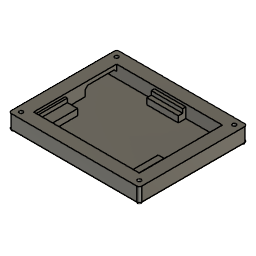
bottom (Autodesk Fusion 360 design; units mm, degrees)
part number: 2026-02-21-15-50-16-128
Autodesk Fusion 360 part; units mm, degrees
sketch "Schizzo1" plane through (0, 0, 0) normal (0, 0, 1) x (1, 0, 0)
  line L0 (0, 0) -> (84, 0)
  line L1 (84, 0) -> (84, 66)
  line L2 (84, 66) -> (0, 66)
  line L3 (0, 66) -> (0, 0)
  line L4 (-10, -10) -> (94, -10)
  line L5 (94, -10) -> (94, 76)
  line L6 (94, 76) -> (-10, 76)
  line L7 (-10, 76) -> (-10, -10)
  circle A0 centre (-5, 71) radius 1.45
  circle A1 centre (-5, -5) radius 1.45
  circle A2 centre (89, -5) radius 1.45
  circle A3 centre (88.5374, 71) radius 1.45
  line L8 (0, 66) -> (84, 66)
  line L9 (84, 66) -> (84, 0)
  line L10 (84, 0) -> (0, 0)
  line L11 (0, 0) -> (0, 66)
  dimension "d1" = 84
  dimension "d2" = 66
  dimension "d3" = 10
  dimension "d4" = 2.9
  dimension "d5" = 2.9
  dimension "d6" = 2.9
  dimension "d7" = 5
  dimension "d8" = 5
  dimension "d9" = 5
  dimension "d10" = 5
  dimension "d11" = 5
  dimension "d12" = 2.9
  dimension "d13" = 5
  dimension "d14" = 5.4626
  constraint horizontal L0
  constraint vertical L1
  constraint horizontal L2
  constraint vertical L3
  constraint coincident L0.start L3.end
  constraint horizontal L8
  constraint vertical L9
  constraint horizontal L10
  constraint vertical L11
  measures "d1" distance of L0.start L0.end
  measures "d2" distance of L0.start L2.end
  measures "d4" diameter of A0
  measures "d5" diameter of A1
  measures "d6" diameter of A2
  measures "d7" distance of L4 A2.centre
  measures "d8" distance of L5 A2.centre
  measures "d9" distance of L4 A1.centre
  measures "d10" distance of L6 A0.centre
  measures "d11" distance of L7 A0.centre
  measures "d12" diameter of A3
  measures "d13" distance of L6 A3.centre
  measures "d14" distance of L5 A3.centre
extrude "Estrusione1" add sketch "Schizzo1" along normal blind 13
sketch "Schizzo2" plane through (0, 0, 0) normal (0, 0, 1) x (1, 0, 0)
  line L0 (0, 0) -> (84, 0)
  line L1 (84, 0) -> (84, 66)
  line L2 (84, 66) -> (0, 66)
  line L3 (0, 66) -> (0, 0)
  constraint horizontal L0
  constraint vertical L1
  constraint horizontal L2
  constraint vertical L3
  constraint coincident L0.start L3.end
extrude "Estrusione2" add sketch "Schizzo2" along normal blind 3
sketch "Sketch3" plane through (-10, 0, 0) normal (-1, 0, 0) x (0, -1, 0)
  line L0 (-76, 0) -> (10, 0)
  line L1 (10, 0) -> (10, 13)
  line L2 (10, 13) -> (-76, 13)
  line L3 (-76, 13) -> (-76, 0)
  line L4 (-66, 3) -> (-41, 3)
  line L5 (-41, 3) -> (-41, 8)
  line L6 (-41, 8) -> (-43, 10)
  line L7 (-43, 10) -> (-64, 10)
  line L8 (-64, 10) -> (-66, 8)
  line L9 (-66, 8) -> (-66, 3)
  constraint horizontal L4
  constraint perpendicular L4 L5
  constraint perpendicular L5 L7
  constraint perpendicular L6 L8
  constraint perpendicular L4 L9
extrude "Extrude3" cut sketch "Sketch3" against normal blind 10 contours L4 L5 L6 L7 L8 L9
fillet "Fillet1" radius 2 4 edges at (94, 33, 0) (42, -10, 0) (-10, 33, 0) (42, 76, 0)
fillet "Fillet2" radius 2 8 edges at (-9.4142, -9.4142, 0.5858) (-10, -10, 7.5) (93.4142, -9.4142, 0.5858) (94, -10, 7.5) (93.4142, 75.4142, 0.5858) (94, 76, 7.5) (-9.4142, 75.4142, 0.5858) (-10, 76, 7.5)
sketch "Sketch4" plane through (0, 0, 3) normal (0, 0, 1) x (-1, 0, 0)
  line L0 (0, -41) -> (0, 0)
  line L1 (0, 0) -> (-84, 0)
  line L2 (-84, 0) -> (-84, -66)
  line L3 (-84, -66) -> (10, -66)
  line L4 (10, -66) -> (10, -41)
  line L5 (10, -41) -> (0, -41)
  line L6 (0, 0) -> (-10, 0)
  line L7 (-10, 0) -> (-10, -25)
  line L8 (-10, -25) -> (0, -25)
  line L9 (0, -25) -> (0, 0)
  constraint horizontal L6
  constraint vertical L7
  constraint horizontal L8
  constraint vertical L9
  constraint coincident L0.end L1.start
extrude "Extrude4" add sketch "Sketch4" along normal blind 5 contours L0 L1 L6 L7 L8 L9
sketch "Sketch5" plane through (0, 0, 3) normal (0, 0, 1) x (-1, 0, 0)
  line L0 (-10, -25) -> (-10, 0)
  line L1 (-10, 0) -> (-84, 0)
  line L2 (-84, 0) -> (-84, -66)
  line L3 (-84, -66) -> (10, -66)
  line L4 (10, -66) -> (10, -41)
  line L5 (10, -41) -> (0, -41)
  line L6 (0, -41) -> (0, -25)
  line L7 (0, -25) -> (-10, -25)
  line L8 (-84, 0) -> (-74, 0)
  line L9 (-74, 0) -> (-74, -25)
  line L10 (-74, -25) -> (-84, -25)
  line L11 (-84, -25) -> (-84, 0)
  constraint horizontal L8
  constraint vertical L9
  constraint horizontal L10
  constraint vertical L11
  constraint coincident L1.end L2.start
extrude "Extrude5" add sketch "Sketch5" along normal blind 5 contours L1 L2 L8 L9 L10 L11
sketch "Sketch6" plane through (0, 0, 3) normal (0, 0, 1) x (-1, 0, 0)
  line L0 (-74, 0) -> (-74, -25)
  line L1 (-74, -25) -> (-84, -25)
  line L2 (-84, -25) -> (-84, -66)
  line L3 (-84, -66) -> (10, -66)
  line L4 (10, -66) -> (10, -41)
  line L5 (10, -41) -> (0, -41)
  line L6 (0, -41) -> (0, -25)
  line L7 (0, -25) -> (-10, -25)
  line L8 (-10, -25) -> (-10, 0)
  line L9 (-10, 0) -> (-74, 0)
  line L10 (-30, -66) -> (-55, -66)
  line L11 (-55, -66) -> (-55, -63.5)
  line L12 (-55, -63.5) -> (-30, -63.5)
  line L13 (-30, -63.5) -> (-30, -66)
  dimension "d29" = 2.5
  constraint horizontal L10
  constraint vertical L11
  constraint horizontal L12
  constraint vertical L13
  constraint coincident L3 L10.start
  measures "d29" distance of L10.start L12.end
extrude "Extrude6" add sketch "Sketch6" along normal blind 8 contours L3 L10 L11 L12 L13
sketch "Sketch7" plane through (0, 0, 3) normal (0, 0, 1) x (-1, 0, 0)
  line L0 (-55, -66) -> (-55, -63.5)
  line L1 (-55, -63.5) -> (-30, -63.5)
  line L2 (-30, -63.5) -> (-30, -66)
  line L3 (-30, -66) -> (10, -66)
  line L4 (10, -66) -> (10, -41)
  line L5 (10, -41) -> (0, -41)
  line L6 (0, -41) -> (0, -25)
  line L7 (0, -25) -> (-10, -25)
  line L8 (-10, -25) -> (-10, 0)
  line L9 (-10, 0) -> (-74, 0)
  line L10 (-74, 0) -> (-74, -25)
  line L11 (-74, -25) -> (-84, -25)
  line L12 (-84, -25) -> (-84, -66)
  line L13 (-84, -66) -> (-55, -66)
  line L14 (-30, -66) -> (-55, -66)
  line L15 (-55, -66) -> (-55, -60)
  line L16 (-55, -60) -> (-30, -60)
  line L17 (-30, -60) -> (-30, -66)
  constraint horizontal L14
  constraint vertical L15
  constraint horizontal L16
  constraint vertical L17
  constraint coincident L2.end L3.start
extrude "Extrude7" add sketch "Sketch7" along normal blind 5 contours L1 L15 L16 L17
sketch "Sketch8" plane through (0, 0, 3) normal (0, 0, 1) x (-1, 0, 0)
  line L0 (-55, -66) -> (-55, -60)
  line L1 (-55, -60) -> (-30, -60)
  line L2 (-30, -60) -> (-30, -66)
  line L3 (-30, -66) -> (10, -66)
  line L4 (10, -66) -> (10, -41)
  line L5 (10, -41) -> (0, -41)
  line L6 (0, -41) -> (0, -25)
  line L7 (0, -25) -> (-10, -25)
  line L8 (-10, -25) -> (-10, 0)
  line L9 (-10, 0) -> (-74, 0)
  line L10 (-74, 0) -> (-74, -25)
  line L11 (-74, -25) -> (-84, -25)
  line L12 (-84, -25) -> (-84, -66)
  line L13 (-84, -66) -> (-55, -66)
  line L14 (-50, 0) -> (-35, 0)
  line L15 (-35, 0) -> (-35, -1.2)
  line L16 (-35, -1.2) -> (-50, -1.2)
  line L17 (-50, -1.2) -> (-50, 0)
  dimension "d34" = 1.2
  constraint horizontal L14
  constraint vertical L15
  constraint horizontal L16
  constraint vertical L17
  constraint coincident L9 L14.start
  measures "d34" distance of L14.start L16.end
extrude "Extrude8" add sketch "Sketch8" along normal blind 8 contours L9 L14 L15 L16 L17
sketch "Sketch9" plane through (0, 0, 3) normal (0, 0, 1) x (-1, 0, 0)
  line L0 (-35, 0) -> (-35, -1.2)
  line L1 (-35, -1.2) -> (-50, -1.2)
  line L2 (-50, -1.2) -> (-50, 0)
  line L3 (-50, 0) -> (-74, 0)
  line L4 (-74, 0) -> (-74, -25)
  line L5 (-74, -25) -> (-84, -25)
  line L6 (-84, -25) -> (-84, -66)
  line L7 (-84, -66) -> (-55, -66)
  line L8 (-55, -66) -> (-55, -60)
  line L9 (-55, -60) -> (-30, -60)
  line L10 (-30, -60) -> (-30, -66)
  line L11 (-30, -66) -> (10, -66)
  line L12 (10, -66) -> (10, -41)
  line L13 (10, -41) -> (0, -41)
  line L14 (0, -41) -> (0, -25)
  line L15 (0, -25) -> (-10, -25)
  line L16 (-10, -25) -> (-10, 0)
  line L17 (-10, 0) -> (-35, 0)
  line L18 (-50, -1.2) -> (-35, -1.2)
  line L19 (-35, -1.2) -> (-35, -3)
  line L20 (-35, -3) -> (-50, -3)
  line L21 (-50, -3) -> (-50, -1.2)
  constraint horizontal L18
  constraint vertical L19
  constraint horizontal L20
  constraint vertical L21
  constraint coincident L1.end L2.start
extrude "Extrude9" add sketch "Sketch9" along normal blind 5 contours L1 L18 L19 L20 L21
sketch "Sketch10" plane through (0, 0, 8) normal (0, 0, 1) x (-1, 0, 0)
  line L0 (-84, -25) -> (-74, -25)
  line L1 (-74, -25) -> (-74, 0)
  line L2 (-74, 0) -> (-84, 0)
  line L3 (-84, 0) -> (-84, -25)
  line L4 (-84, 0) -> (-81.8, 0)
  line L5 (-81.8, 0) -> (-81.8, -25)
  line L6 (-81.8, -25) -> (-84, -25)
  line L7 (-84, -25) -> (-84, 0)
  dimension "d39" = 2.2
  constraint horizontal L4
  constraint vertical L5
  constraint horizontal L6
  constraint vertical L7
  constraint coincident L0 L5.end
  constraint coincident L2.end L3.start
  measures "d39" distance of L2.end L4.end
extrude "Extrude10" add sketch "Sketch10" along normal blind 3 contours L0 L2 L3 L4 L5 L6 L7
sketch "Sketch11" plane through (0, 0, 8) normal (0, 0, 1) x (-1, 0, 0)
  line L0 (0, -25) -> (0, 0)
  line L1 (0, 0) -> (-10, 0)
  line L2 (-10, 0) -> (-10, -25)
  line L3 (-10, -25) -> (0, -25)
  line L4 (0, 0) -> (-1.8, 0)
  line L5 (-1.8, 0) -> (-1.8, -25)
  line L6 (-1.8, -25) -> (0, -25)
  line L7 (0, -25) -> (0, 0)
  dimension "d42" = 1.8
  constraint horizontal L4
  constraint vertical L5
  constraint horizontal L6
  constraint vertical L7
  constraint coincident L0.end L1.start
  measures "d42" distance of L0.end L4.end
extrude "Extrude11" add sketch "Sketch11" along normal blind 3 contours L0 L1 L3 L4 L5 L6 L7
extrude "Extrude12" cut 1 faces at (4.5333, 16.6667, 8) along direction (0, 0, -1) blind 0.1
extrude "Extrude13" cut 1 faces at (79.2, 8.3333, 8) along direction (0, 0, -1) blind 0.1
extrude "Extrude14" cut 1 faces at (46.6667, 61.1667, 8) along direction (0, 0, -1) blind 0.1
extrude "Extrude15" cut 1 faces at (45, 2.4, 8) along direction (0, 0, -1) blind 0.1
